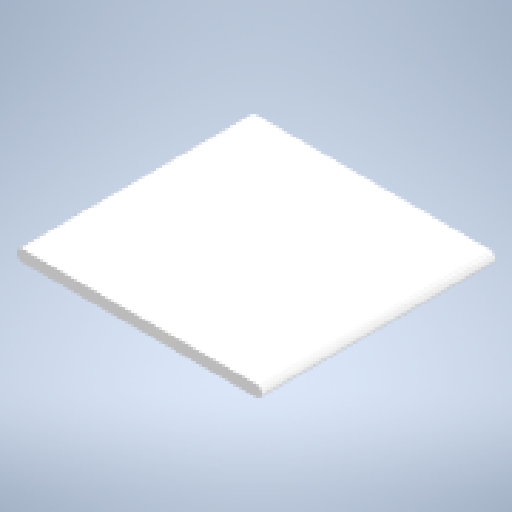
# Autodesk Inventor part: Schaufelplatten
Saved by Autodesk Inventor 2024.4 (Build 284460000, 460)
## iProperties
Created: 2026-01-10
Part Number: Schaufelplatten
Material: PVC, hart
Description: Schaufelplatten
Document SubType Name: Modeling
Designer: Philf
Mass: 304.063 g
Surface Area: 526.403 cm^2
Volume: 235.708 cm^3
Density: 1.29 g/cm^3
Appearance: Glatt - Weiß
Autodesk Inventor part; units mm, degrees
ref_plane "YZ Plane" through (0, 0, 0) normal (1, 0, 0) x (0, 1, 0)
ref_plane "XZ Plane" through (0, 0, 0) normal (0, 1, 0) x (-1, 0, 0)
ref_plane "XY Plane" through (0, 0, 0) normal (0, 0, 1) x (1, 0, 0)
sketch "Skizze1" plane through (0, 0, 0) normal (0, 1, 0) x (-1, 0, 0)
  line L0 (0, 0) -> (220, 0)
  line L1 (220, 0) -> (220, -10)
  line L2 (220, -10) -> (0, -10)
  line L3 (0, -10) -> (0, 0)
  circle A0 centre (5, -5) radius 5
  circle A1 centre (215, -5) radius 5
  point P0 (5, -10)
  point P1 (215, -10)
  point P2 (215, 0)
  point P3 (5, 0)
  dimension "d0" = 220
  dimension "d1" = 10
  constraints: 8 end point, 6 tangent, 2 centre point, 2 perpendicular, 1 horizontal, 1 vertical
  measures "d0" distance of L0.start L0.end
  measures "d1" distance of L0.end L1.end
extrude "Extrusion1" add sketch "Skizze1" along normal blind 200 contours L0 A1 L2 A0 | A0 | A1
equation "\"d0\" = nutlange + radius"
equation "\"nutlange\" = 210"
equation "\"radius\" = 10"
